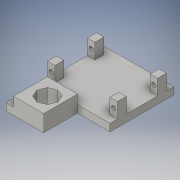
# Autodesk Inventor part: leftside
Saved by Autodesk Inventor 2016 (Build 200138000, 138)
## iProperties
Created: 2015-04-28
Part Number: leftside
Material: Generic
Document SubType Name: Modeling
Designer: Jacob Kennedy
Density: 1 g/cm^3
Appearance: Default
Author: Jacob Kennedy
Autodesk Inventor part; units mm, degrees
ref_plane "YZ Plane" through (0, 0, 0) normal (1, 0, 0) x (0, 1, 0)
ref_plane "XZ Plane" through (0, 0, 0) normal (0, 1, 0) x (-1, 0, 0)
ref_plane "XY Plane" through (0, 0, 0) normal (0, 0, 1) x (1, 0, 0)
sketch "Sketch1" plane through (0, 0, 0) normal (0, 1, 0) x (-1, 0, 0)
  line L0 (10.0298, 10.8298) -> (-22.0758, 10.8298)
  line L1 (-22.0758, 10.8298) -> (-22.0758, -18.1453)
  line L2 (-22.0758, -18.1453) -> (10.0298, -18.1453)
  line L3 (10.0298, -18.1453) -> (10.0298, 10.8298)
  line L4 (10.0298, 10.8298) -> (0.708, 10.8298)
  line L5 (10.0298, 4.4798) -> (10.0298, 10.8298)
  line L6 (10.0298, -18.1453) -> (0.708, -18.1453)
  line L7 (10.0298, -11.954) -> (10.0298, -18.1453)
  line L8 (-22.0758, 4.4798) -> (-22.0758, -11.954)
  line L9 (-4.274, -9.9621) -> (-10.5532, -12.6713)
  line L10 (-10.5532, -12.6713) -> (-16.9089, -10.147)
  line L11 (-16.9089, -10.147) -> (-19.6181, -3.8679)
  line L12 (-19.6181, -3.8679) -> (-17.0938, 2.4878)
  line L13 (-17.0938, 2.4878) -> (-10.8147, 5.1971)
  line L14 (-10.8147, 5.1971) -> (-4.459, 2.6728)
  line L15 (-4.459, 2.6728) -> (-1.7498, -3.6063)
  line L16 (-1.7498, -3.6063) -> (-4.274, -9.9621)
  point P0 (0, 0)
  point P1 (-10.6839, -3.7371)
  dimension "d0" = 28.975
  dimension "d1" = 32.1056
  constraints: 34 end point, 3 horizontal, 2 parallel, 1 perpendicular, 1 point on line, 17 other
  measures "d0" distance of L2.end L0.start
  measures "d1" distance of L1.end L2.end
extrude "Extrusion1" add sketch "Sketch1" along normal blind 14.224
sketch "Sketch2" plane through (0, 0, 0) normal (0, -1, 0) x (1, 0, 0)
  line L0 (-10.0298, -18.1453) -> (-10.0298, 10.8298) projected
  line L1 (-10.0298, -18.1453) -> (49.7745, -18.1453)
  line L2 (49.7745, -18.1453) -> (49.7745, -24.4953)
  line L3 (49.7745, -24.4953) -> (-10.0298, -24.4953)
  line L4 (-10.0298, -24.4953) -> (-10.0298, -18.1453)
  line L5 (-10.0298, -24.4953) -> (49.7745, -24.4953)
  line L6 (49.7745, -24.4953) -> (49.7745, -72.7553)
  line L7 (49.7745, -72.7553) -> (-10.0298, -72.7553)
  line L8 (-10.0298, -72.7553) -> (-10.0298, -24.4953)
  line L9 (-10.0298, -24.4953) -> (-3.6798, -24.4953)
  line L10 (-3.6798, -24.4953) -> (-3.6798, -32.1153)
  line L11 (-3.6798, -32.1153) -> (-10.0298, -32.1153)
  line L12 (-10.0298, -32.1153) -> (-10.0298, -24.4953)
  line L13 (49.7745, -24.4953) -> (43.4245, -24.4953)
  line L14 (43.4245, -24.4953) -> (43.4245, -32.1153)
  line L15 (43.4245, -32.1153) -> (49.7745, -32.1153)
  line L16 (49.7745, -32.1153) -> (49.7745, -24.4953)
  line L17 (49.7745, -72.7553) -> (-10.0298, -72.7553)
  line L18 (-10.0298, -72.7553) -> (-10.0298, -66.4053)
  line L19 (-10.0298, -66.4053) -> (49.7745, -66.4053)
  line L20 (49.7745, -66.4053) -> (49.7745, -72.7553)
  line L21 (-10.0298, -66.4053) -> (-3.6798, -66.4053)
  line L22 (-3.6798, -66.4053) -> (-3.6798, -58.7853)
  line L23 (-3.6798, -58.7853) -> (-10.0298, -58.7853)
  line L24 (-10.0298, -58.7853) -> (-10.0298, -66.4053)
  line L25 (49.7745, -66.4053) -> (43.4245, -66.4053)
  line L26 (43.4245, -66.4053) -> (43.4245, -58.7853)
  line L27 (43.4245, -58.7853) -> (49.7745, -58.7853)
  line L28 (49.7745, -58.7853) -> (49.7745, -66.4053)
  point P0 (0, 0)
  dimension "d8" = 59.8043
  dimension "d9" = 6.35
  dimension "d10" = 48.26
  dimension "d11" = 6.35
  dimension "d12" = 7.62
  dimension "d13" = 6.35
  dimension "d14" = 6.35
  dimension "d15" = 6.35
  dimension "d16" = 7.62
  constraints: 56 end point, 14 parallel, 7 horizontal, 7 perpendicular, 3 point on line
  measures "d8" distance of L2.end L3.end
  measures "d9" distance of L1.end L2.end
  measures "d10" distance of L7.end L3.end
  measures "d11" distance of L10.end L11.end
  measures "d12" distance of L9.end L10.end
  measures "d13" distance of L15.end L14.end
  measures "d14" distance of L17.end L18.end
  measures "d15" distance of L23.end L22.end
  measures "d16" distance of L22.end L21.end
extrude "Extrusion2" add sketch "Sketch2" against normal blind 6.35
sketch "Sketch3" plane through (0, 6.35, 0) normal (0, 1, 0) x (1, 0, 0)
  line L0 (-10.0298, -10.8298) -> (-10.0298, 72.7553) projected
  line L1 (49.7745, 18.1453) -> (49.7745, 72.7553) projected
  line L2 (-10.0298, 72.7553) -> (49.7745, 72.7553)
  line L3 (49.7745, 72.7553) -> (49.7745, 66.4053)
  line L4 (49.7745, 66.4053) -> (-10.0298, 66.4053)
  line L5 (-10.0298, 66.4053) -> (-10.0298, 72.7553)
  line L6 (-10.0298, 66.4053) -> (-3.6798, 66.4053)
  line L7 (-3.6798, 66.4053) -> (-3.6798, 58.7853)
  line L8 (-3.6798, 58.7853) -> (-10.0298, 58.7853)
  line L9 (-10.0298, 58.7853) -> (-10.0298, 66.4053)
  line L10 (49.7745, 66.4053) -> (43.4245, 66.4053)
  line L11 (43.4245, 66.4053) -> (43.4245, 58.7853)
  line L12 (43.4245, 58.7853) -> (49.7745, 58.7853)
  line L13 (49.7745, 58.7853) -> (49.7745, 66.4053)
  line L14 (22.0758, 18.1453) -> (-10.0298, 18.1453) projected
  line L15 (-10.0298, 18.1453) -> (-3.6798, 18.1453)
  line L16 (49.7745, 18.1453) -> (43.4245, 18.1453)
  line L17 (-10.0298, 18.1453) -> (49.7745, 18.1453)
  line L18 (49.7745, 24.4953) -> (-10.0298, 24.4953)
  line L19 (-10.0298, 24.4953) -> (-10.0298, 18.1453)
  line L20 (-10.0298, 24.4953) -> (-3.6798, 24.4953)
  line L21 (-3.6798, 24.4953) -> (-3.6798, 32.1487)
  line L22 (-3.6798, 32.1487) -> (-10.0298, 32.1487)
  line L23 (-10.0298, 32.1487) -> (-10.0298, 24.4953)
  line L24 (49.7745, 24.4953) -> (43.4245, 24.4953)
  line L25 (43.4245, 24.4953) -> (43.4245, 32.1487)
  line L26 (43.4245, 32.1487) -> (49.7745, 32.1487)
  line L27 (49.7745, 32.1487) -> (49.7745, 24.4953)
  point P0 (0, 0)
  dimension "d19" = 6.35
  dimension "d20" = 6.35
  dimension "d21" = 7.62
  dimension "d22" = 6.35
  dimension "d23" = 7.62
  dimension "d26" = 6.35
  constraints: 50 end point, 11 parallel, 8 horizontal, 5 perpendicular, 2 point on line
  measures "d19" distance of L4.end L0.end
  measures "d20" distance of L7.end L8.end
  measures "d21" distance of L6.end L7.end
  measures "d22" distance of L12.end L11.end
  measures "d23" distance of L11.end L10.end
  measures "d26" distance of L18.end L14.end
extrude "Extrusion3" add sketch "Sketch3" along normal blind 13.0048 contours L0 L22 L21 L18 | L0 L4 L7 L8 | L25 L26 L1 L18 | L4 L1 L12 L11
sketch "Sketch4" plane through (-10.0298, 0, 10.8298) normal (0, 0, 1) x (1, 0, 0)
  line L0 (32.1056, 14.224) -> (0, 14.224) projected
  line L1 (6.35, 6.35) -> (6.35, 19.3548) projected
  line L2 (0, 14.224) -> (6.35, 14.224)
  line L3 (6.35, 14.224) -> (6.35, 6.35)
  line L4 (6.35, 6.35) -> (0, 6.35)
  line L5 (0, 6.35) -> (0, 14.224)
  point P0 (10.0298, 0)
  constraints: 8 end point, 2 parallel, 1 horizontal, 1 perpendicular
extrude "Extrusion4" cut sketch "Sketch4" along normal mid plane 64.7827
sketch "Sketch5" plane through (-3.6798, 6.35, -66.4053) normal (0, 0, -1) x (-1, 0, 0)
  line L0 (6.35, 13.0048) -> (0, 0)
  line L1 (0, 0) -> (0, 13.0048) projected
  line L2 (0, 0) -> (0, 13.0048)
  line L3 (0, 0) -> (6.35, 0) projected
  line L4 (0, 13.0048) -> (6.35, 0)
  line L5 (-53.4543, 0) -> (-53.4543, 13.0048) projected
  line L6 (-53.4543, 13.0048) -> (-47.2741, 0)
  line L7 (-47.2741, 13.0048) -> (-53.4543, 0)
  circle A0 centre (3.175, 6.5024) radius 1.8796
  circle A1 centre (-50.3642, 6.5024) radius 1.8796
  point P0 (-3.6798, -6.35)
  dimension "d31" = 3.7592
  dimension "d32" = 3.7592
  constraints: 10 end point, 2 centre point, 2 midpoint, 1 collinear
  measures "d31" diameter of A0
  measures "d32" diameter of A1
extrude "Extrusion5" cut sketch "Sketch5" along normal mid plane 183.8452 contours A0 L4 L0 | L0 L4 A0 | L4 A0 L0 | L0 A0 L4 | A1 L6 L7 | L7 L6 A1 | A1 L7 L6 | L7 A1 L6
body "Solid1"
